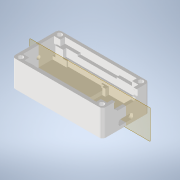
# Autodesk Inventor part: Gehäuse
Saved by Autodesk Inventor 2022 (Build 260153000, 153)
## iProperties
Created: 2021-11-08
Part Number: Gehäuse
Material: Generisch
Document SubType Name: Modeling
Designer: lukas
Density: 1 g/cm^3
Appearance: Vorgabe
Author: lukas
Autodesk Inventor part; units mm, degrees
ref_plane "YZ Plane" through (0, 0, 0) normal (1, 0, 0) x (0, 1, 0)
ref_plane "XZ Plane" through (0, 0, 0) normal (0, 1, 0) x (-1, 0, 0)
ref_plane "XY Plane" through (0, 0, 0) normal (0, 0, 1) x (1, 0, 0)
sketch "Skizze1" plane through (0, 0, 0) normal (0, 1, 0) x (-1, 0, 0)
  line L0 (0, 0) -> (58, 0)
  line L1 (58, 0) -> (58, -30)
  line L2 (58, -30) -> (0, -30)
  line L3 (0, -30) -> (0, 0)
  dimension "d0" = 30
  dimension "d1" = 58
  constraints: 8 end point, 2 parallel, 1 horizontal, 1 perpendicular
  measures "d0" distance between parallel lines of L0 L2
  measures "d1" distance of L1.end L2.end
extrude "Extrusion1" add sketch "Skizze1" along normal blind 2
sketch "Skizze2" plane through (0, 2, 0) normal (0, 1, 0) x (1, 0, 0)
  line L0 (0, 30) -> (-58, 30) projected
  line L1 (-58, 30) -> (-58, 0) projected
  line L2 (-58, 0) -> (0, 0) projected
  line L3 (0, 0) -> (0, 30) projected
  line L4 (-56, 28) -> (-2, 28)
  line L5 (-2, 28) -> (-2, 2)
  line L6 (-2, 2) -> (-56, 2)
  line L7 (-56, 2) -> (-56, 28)
  dimension "d4" = 2
  constraints: 8 end point, 3 other
  measures "d4" distance between parallel lines of L0 L4
extrude "Extrusion2" add sketch "Skizze2" along normal blind 13.7
ref_plane "Arbeitsebene1" through (-56, 2, -15) normal (0, 0, 1) x (1, 0, 0)
ref_plane "Arbeitsebene2" through (-22.61, 3.28, -21) normal (0, -1, 0) x (1, 0, 0)
sketch "Skizze6" plane through (0, 2, 0) normal (0, 1, 0) x (1, 0, 0)
  line L0 (-13, 15.5) -> (-2, 15.5) projected
  line L1 (-2, 15.5) -> (-2, 25.925) projected
  line L2 (-2, 25.925) -> (-49.2, 25.925) projected
  line L3 (-49.2, 25.925) -> (-49.2, 4.075) projected
  line L4 (-49.2, 4.075) -> (-2, 4.075) projected
  line L5 (-2, 4.075) -> (-2, 14.5) projected
  line L6 (-2, 14.5) -> (-13, 14.5) projected
  line L7 (-13, 14.5) -> (-13, 15.5) projected
  line L8 (-24.31, 7.3) -> (-24.31, 22.7) projected
  line L9 (-24.31, 22.7) -> (-17.4058, 22.7) projected
  line L10 (-17.4058, 22.7) -> (-16.0058, 21.3) projected
  line L11 (-16.0058, 21.3) -> (-7.41, 21.3) projected
  line L12 (-7.41, 8.7) -> (-16.0058, 8.7) projected
  line L13 (-16.0058, 8.7) -> (-17.4058, 7.3) projected
  line L14 (-17.4058, 7.3) -> (-24.31, 7.3) projected
  line L15 (-48.9344, 26.05) -> (-46.9344, 26.05)
  line L16 (-46.9344, 26.05) -> (-46.9344, 3.95)
  line L17 (-46.9344, 3.95) -> (-48.9344, 3.95)
  line L18 (-48.9344, 3.95) -> (-48.9344, 26.05)
  line L19 (-0.8, 14.3) -> (-11.8, 14.3)
  line L20 (-11.8, 14.3) -> (-11.8, 15.7)
  line L21 (-11.8, 15.7) -> (-0.8, 15.7)
  line L22 (-0.8, 15.7) -> (-0.8, 2.875)
  line L23 (-0.8, 2.875) -> (-50.4, 2.875)
  line L24 (-50.4, 2.875) -> (-50.4, 27.125)
  line L25 (-50.4, 27.125) -> (-0.8, 27.125)
  line L26 (-0.8, 27.125) -> (-0.8, 14.3)
  line L27 (-48.2, 24.925) -> (-3, 24.925)
  line L28 (-3, 24.925) -> (-3, 16.5)
  line L29 (-3, 16.5) -> (-14, 16.5)
  line L30 (-14, 16.5) -> (-14, 13.5)
  line L31 (-14, 13.5) -> (-3, 13.5)
  line L32 (-3, 13.5) -> (-3, 5.075)
  line L33 (-3, 5.075) -> (-48.2, 5.075)
  line L34 (-48.2, 5.075) -> (-48.2, 24.925)
  line L35 (-13.5, 6.075) -> (-13.5, 23.925) projected
  line L36 (-2, 6.075) -> (-13.5, 6.075) projected
  line L37 (-13.5, 23.925) -> (-2, 23.925) projected
  line L38 (-2, 23.925) -> (-2, 6.075) projected
  line L39 (-3, 5.075) -> (-2, 5.075)
  line L40 (-2, 2) -> (-2, 28) projected
  line L41 (-3, 24.925) -> (-2, 24.925)
  line L42 (-2, 2) -> (-2, 28) projected
  line L43 (-46.9344, 3.95) -> (-46.9344, 2.875)
  line L44 (-46.9344, 26.05) -> (-46.9344, 27.125)
  line L45 (-50.4, 27.125) -> (-46.9344, 27.125)
  line L46 (-46.9344, 27.125) -> (-46.9344, 26.25)
  line L47 (-46.9344, 26.25) -> (-50.4, 26.25)
  line L48 (-50.4, 26.25) -> (-50.4, 27.125)
  line L49 (-50.4, 2.875) -> (-46.9344, 2.875)
  line L50 (-46.9344, 2.875) -> (-46.9344, 3.75)
  line L51 (-46.9344, 3.75) -> (-50.4, 3.75)
  line L52 (-50.4, 3.75) -> (-50.4, 2.875)
  line L53 (-68, 2.495) -> (-68, 27.05)
  line L54 (-56, 28) -> (-56, 2) projected
  line L55 (-50.4, 27.125) -> (-56, 27.125)
  line L56 (-50.4, 2.875) -> (-56, 2.875)
  line L57 (-2, 28) -> (-56, 28) projected
  line L58 (-50.4, 27.125) -> (-2, 27.125)
  line L59 (-2, 27.125) -> (-2, 28)
  line L60 (-2, 28) -> (-50.4, 28)
  line L61 (-50.4, 28) -> (-50.4, 27.125)
  line L62 (-56, 2) -> (-2, 2) projected
  line L63 (-50.4, 3.75) -> (-2, 3.75)
  line L64 (-2, 3.75) -> (-2, 2)
  line L65 (-2, 2) -> (-50.4, 2)
  line L66 (-50.4, 2) -> (-50.4, 3.75)
  line L67 (-54.3, 2) -> (-49.3, 2)
  line L68 (-49.3, 2) -> (-49.3, 6)
  line L69 (-49.3, 6) -> (-54.3, 6)
  line L70 (-54.3, 6) -> (-54.3, 2)
  line L71 (-54.3, 28) -> (-49.3, 28)
  line L72 (-49.3, 28) -> (-49.3, 24)
  line L73 (-49.3, 24) -> (-54.3, 24)
  line L74 (-54.3, 24) -> (-54.3, 28)
  line L75 (-54.3, 6) -> (-46.9344, 6)
  line L76 (-46.9344, 6) -> (-46.9344, 2)
  line L77 (-46.9344, 2) -> (-54.3, 2)
  line L78 (-54.3, 2) -> (-54.3, 6)
  line L79 (-54.3, 24) -> (-46.9344, 24)
  line L80 (-46.9344, 24) -> (-46.9344, 28)
  line L81 (-46.9344, 28) -> (-54.3, 28)
  line L82 (-54.3, 28) -> (-54.3, 24)
  point P0 (0, 0)
  point P1 (-2, 11.83)
  point P2 (-2, 18.17)
  point P3 (-2, 2.875)
  point P4 (-46.9344, 5.075)
  point P5 (-46.9344, 24.925)
  point P6 (-2, 27.125)
  point P7 (-54.3, 2.875)
  point P8 (-50.4, 6)
  point P9 (-49.3, 3.75)
  point P10 (-50.4, 24)
  point P11 (-49.3, 26.25)
  point P12 (-54.3, 27.125)
  point P13 (-50.4, 24)
  point P14 (-50.4, 6)
  dimension "d26" = 2
  dimension "d27" = 1
  dimension "d53" = 0.1
  dimension "d54" = 5
  dimension "d55" = 4
  dimension "d56" = 4
  constraints: 118 end point, 19 parallel, 14 point on line, 12 perpendicular, 10 horizontal, 14 other
  measures "d26" distance of L16.end L17.end
  measures "d27" distance between parallel lines of L2 L27
  measures "d53" distance between parallel lines of L3 L68
  measures "d54" distance between parallel lines of L68 L70
  measures "d55" distance between parallel lines of L62 L69
  measures "d56" distance of L71.end L72.end
ref_plane "Arbeitsebene3" through (-49.2, 7, -25.925) normal (0, -1, 0) x (1, 0, 0)
extrude "Extrusion6" add sketch "Skizze6" along normal blind 5 contours L41 L27 L16 L2 L1 | L2 L16 L44 L25 L40 | L25 L80 L57 L40 | L5 L4 L16 L33 L39 | L16 L27 L34 L79 L18 L2 | L2 L18 L15 L16 | L16 L79 L34 L27 | L40 L62 L76 L23 | L23 L43 L63 L40 | L44 L47 L72 L25 | L25 L72 L57 L80 | L40 L63 L43 L16 L4 | L18 L79 L3 L2 | L2 L3 L79 L72 L47 L44 L15 L18 | L76 L62 L68 L23 | L23 L68 L51 L43 | L72 L47 L24 L25 | L25 L61 L57 L72 | L16 L17 L18 L4 | L4 L18 L75 L34 L33 L16 | L33 L34 L75 L16 | L68 L62 L66 L23 | L23 L24 L51 L68 | L51 L68 L75 L3 L4 L18 L17 L43 | L24 L73 L74 L55 | L55 L74 L57 L61 | L72 L73 L24 L47 | L4 L3 L75 L18 | L56 L70 L69 L24 | L66 L62 L70 L56 | L51 L24 L69 L68
sketch "Skizze9" plane through (-50.4, 7, -27.125) normal (0, 1, 0) x (1, 0, 0)
  line L0 (37.4, -11.625) -> (48.4, -11.625) projected
  line L1 (48.4, -11.625) -> (48.4, -1.2) projected
  line L2 (48.4, -1.2) -> (1.2, -1.2) projected
  line L3 (1.2, -1.2) -> (1.2, -23.05) projected
  line L4 (1.2, -23.05) -> (48.4, -23.05) projected
  line L5 (48.4, -23.05) -> (48.4, -12.625) projected
  line L6 (48.4, -12.625) -> (37.4, -12.625) projected
  line L7 (37.4, -12.625) -> (37.4, -11.625) projected
  line L8 (1.1, -1.1) -> (48.5, -1.1)
  line L9 (48.5, -1.1) -> (48.5, -11.725)
  line L10 (48.5, -11.725) -> (37.5, -11.725)
  line L11 (37.5, -11.725) -> (37.5, -12.525)
  line L12 (37.5, -12.525) -> (48.5, -12.525)
  line L13 (48.5, -12.525) -> (48.5, -23.15)
  line L14 (48.5, -23.15) -> (1.1, -23.15)
  line L15 (1.1, -23.15) -> (1.1, -1.1)
  line L16 (3.4656, -21.125) -> (-3.9, -21.125) projected
  line L17 (-3.9, -21.125) -> (-3.9, -25.125) projected
  line L18 (48.4, -25.125) -> (-3.9, -25.125) projected
  line L19 (48.4, -22.05) -> (48.4, -25.125) projected
  line L20 (48.4, -22.05) -> (3.4656, -22.05) projected
  line L21 (3.4656, -22.05) -> (3.4656, -21.125) projected
  line L22 (3.4656, -2.2) -> (48.4, -2.2) projected
  line L23 (48.4, 0.875) -> (48.4, -2.2) projected
  line L24 (-3.9, 0.875) -> (48.4, 0.875) projected
  line L25 (-3.9, 0.875) -> (-3.9, -3.125) projected
  line L26 (-3.9, -3.125) -> (3.4656, -3.125) projected
  line L27 (3.4656, -3.125) -> (3.4656, -2.2) projected
  point P0 (50.4, -27.125)
  point P1 (1.1, -3.125)
  point P2 (48.4, -1.1)
  point P3 (48.4, -23.15)
  point P4 (1.1, -21.125)
  dimension "d41" = 0.1
  constraints: 16 end point, 7 other
  measures "d41" distance between parallel lines of L2 L8
extrude "Extrusion9" add sketch "Skizze9" along normal blind 5 contours L8 L15 L26 L25 L24 L23 | L19 L18 L17 L16 L15 L14
sketch "Skizze13" plane through (-50.4, 12, -27.125) normal (0, 1, 0) x (1, 0, 0)
  line L0 (48.4, -25.125) -> (-3.9, -25.125) projected
  line L1 (48.4, -23.15) -> (48.4, -25.125) projected
  line L2 (48.4, -23.15) -> (1.1, -23.15) projected
  line L3 (1.1, -23.15) -> (1.1, -21.125) projected
  line L4 (1.1, -21.125) -> (-3.9, -21.125) projected
  line L5 (-3.9, -21.125) -> (-3.9, -25.125) projected
  line L6 (-3.9, -3.125) -> (1.1, -3.125) projected
  line L7 (1.1, -3.125) -> (1.1, -1.1) projected
  line L8 (1.1, -1.1) -> (48.4, -1.1) projected
  line L9 (48.4, 0.875) -> (48.4, -1.1) projected
  line L10 (-3.9, 0.875) -> (48.4, 0.875) projected
  line L11 (-3.9, 0.875) -> (-3.9, -3.125) projected
  line L12 (48.4, -25.125) -> (-3.9, -25.125) projected
  line L13 (48.4, -23.15) -> (1.1, -23.15) projected
  line L14 (33.4, -25.125) -> (8.4, -25.125)
  line L15 (8.4, -25.125) -> (8.4, -23.15)
  line L16 (8.4, -23.15) -> (33.4, -23.15)
  line L17 (33.4, -23.15) -> (33.4, -25.125)
  line L18 (-3.9, 0.875) -> (48.4, 0.875) projected
  line L19 (33.4, -1.1) -> (8.4, -1.1)
  line L20 (8.4, -1.1) -> (8.4, 0.875)
  line L21 (8.4, 0.875) -> (33.4, 0.875)
  line L22 (33.4, 0.875) -> (33.4, -1.1)
  point P0 (50.4, -27.125)
  point P1 (8.4, 0.875)
  point P2 (8.4, -1.1)
  point P3 (33.4, -25.125)
  point P4 (33.4, -23.15)
  point P5 (8.4, -23.15)
  point P6 (8.4, -25.125)
  dimension "d81" = 25
  dimension "d82" = 15
  constraints: 16 end point, 6 point on line, 4 parallel, 2 horizontal, 2 perpendicular
  measures "d81" distance of L15.end L16.end
  measures "d82" distance between parallel lines of L1 L17
extrude "Extrusion13" cut sketch "Skizze13" against normal blind 1 contours L0 L15 L2 L17 | L10 L22 L8 L20
sketch "Skizze14" plane through (-58, 0, -30) normal (-1, 0, 0) x (0, 0, 1)
  line L0 (0, 0) -> (30, 0) projected
  line L1 (30, 0) -> (30, 15.7) projected
  line L2 (0, 15.7) -> (30, 15.7) projected
  line L3 (0, 0) -> (0, 15.7) projected
  circle A0 centre (15, 8.7) radius 1.275
  line L4 (0, 15.7) -> (30, 15.7) projected
  point P0 (15, 15.7)
  dimension "d85" = 2.55
  dimension "d86" = 7
  constraints: 1 centre point, 1 midpoint, 1 vertical alignment
  measures "d85" diameter of A0
  measures "d86" distance from line of L2 A0.centre
extrude "Extrusion14" cut sketch "Skizze14" against normal blind 3 contours A0
sketch "Skizze15" plane through (0, 0, 0) normal (1, 0, 0) x (0, 0, -1)
  line L0 (7.5, 14.875) -> (7.5, 12.3966) projected
  arc A0 (8.3, 15.675) -> (7.5, 14.875) centre (8.3, 14.875) ccw projected
  arc A1 (7.5, 12.3966) -> (8.0647, 11.6319) centre (8.3, 12.3966) ccw projected
  line L1 (8.0647, 11.6319) -> (8.612, 11.4636) projected
  arc A2 (8.7489, 11.375) -> (8.612, 11.4636) centre (8.5237, 11.1768) ccw projected
  line L2 (8.7489, 11.375) -> (9.61, 10.3965) projected
  arc A3 (9.61, 10.3965) -> (10.2106, 10.125) centre (10.2106, 10.925) ccw projected
  line L3 (10.2106, 10.125) -> (19.7894, 10.125) projected
  arc A4 (19.7894, 10.125) -> (20.39, 10.3965) centre (19.7894, 10.925) ccw projected
  line L4 (21.2511, 11.375) -> (20.39, 10.3965) projected
  arc A5 (21.388, 11.4636) -> (21.2511, 11.375) centre (21.4763, 11.1768) ccw projected
  line L5 (21.388, 11.4636) -> (21.9353, 11.6319) projected
  arc A6 (21.9353, 11.6319) -> (22.5, 12.3966) centre (21.7, 12.3966) ccw projected
  line L6 (22.5, 12.3966) -> (22.5, 14.875) projected
  arc A7 (22.5, 14.875) -> (21.7, 15.675) centre (21.7, 14.875) ccw projected
  line L7 (8.3, 15.675) -> (21.7, 15.675) projected
  line L8 (21.229, 11.5716) -> (21.2224, 11.5696)
  line L9 (7.35, 12.3966) -> (7.35, 14.875)
  arc A8 (8.3, 15.825) -> (7.35, 14.875) centre (8.3, 14.875) ccw
  line L10 (8.3, 15.825) -> (21.7, 15.825)
  arc A9 (22.65, 14.875) -> (21.7, 15.825) centre (21.7, 14.875) ccw
  line L11 (22.65, 14.875) -> (22.65, 12.3966)
  arc A10 (21.9794, 11.4886) -> (22.65, 12.3966) centre (21.7, 12.3966) ccw
  line L12 (21.9794, 11.4886) -> (21.4322, 11.3202)
  arc A11 (21.4322, 11.3202) -> (21.3637, 11.2759) centre (21.4763, 11.1768) ccw
  line L13 (21.3637, 11.2759) -> (20.5026, 10.2974)
  arc A12 (19.7894, 9.975) -> (20.5026, 10.2974) centre (19.7894, 10.925) ccw
  line L14 (19.7894, 9.975) -> (10.2106, 9.975)
  arc A13 (9.4974, 10.2974) -> (10.2106, 9.975) centre (10.2106, 10.925) ccw
  line L15 (9.4974, 10.2974) -> (8.6363, 11.2759)
  arc A14 (8.6363, 11.2759) -> (8.5678, 11.3202) centre (8.5237, 11.1768) ccw
  line L16 (8.5678, 11.3202) -> (8.0206, 11.4886)
  arc A15 (7.35, 12.3966) -> (8.0206, 11.4886) centre (8.3, 12.3966) ccw
  point P0 (0, 0)
  dimension "d124" = 0.15
  constraints: 18 end point, 16 point on circle, 8 centre point, 15 other
  measures "d124" distance between parallel lines of L0 L9
extrude "Extrusion15" cut sketch "Skizze15" against normal blind 3 contours A0 L7 A7 L6 A6 L5 A5 L4 A4 L3 A3 L2 A2 L1 A1 L0 | L9 A8 L10 A9 L11 A10 L12 A11 L13 A12 L14 A13 L15 A14 L16 A15
sketch "Skizze17" plane through (-56, 2, -2) normal (1, 0, 0) x (0, 0, -1)
  line L0 (26, 0) -> (26, 13.7) projected
  line L1 (0, 13.7) -> (26, 13.7) projected
  line L2 (0, 0) -> (0, 13.7) projected
  line L3 (26, 0) -> (0, 0) projected
  line L4 (0, 13.7) -> (26, 13.7) projected
  line L5 (0, 13.7) -> (3, 13.7)
  line L6 (3, 13.7) -> (3, 9.5)
  line L7 (3, 9.5) -> (0, 9.5)
  line L8 (0, 9.5) -> (0, 13.7)
  line L9 (26, 4.5) -> (26, 13.7) projected
  line L10 (26, 13.7) -> (23, 13.7)
  line L11 (23, 13.7) -> (23, 9.5)
  line L12 (23, 9.5) -> (26, 9.5)
  line L13 (26, 9.5) -> (26, 13.7)
  point P0 (-2, -2)
  point P1 (26, 9.5)
  point P2 (0, 9.5)
  dimension "d98" = 3
  dimension "d99" = 4.2
  dimension "d100" = 3
  dimension "d101" = 4.2
  constraints: 16 end point, 4 parallel, 2 horizontal, 2 perpendicular
  measures "d98" distance of L6.end L7.end
  measures "d99" distance of L5.end L6.end
  measures "d100" distance of L12.end L11.end
  measures "d101" distance of L11.end L10.end
extrude "Extrusion17" add sketch "Skizze17" along normal blind 4 contours L12 L11 L1 L0 | L2 L1 L6 L7
chamfer "Fase1" distance 3 angle 45 2 edges at (-55.15, 11.5, -2) (-55.15, 11.5, -28)
sketch "Skizze18" plane through (0, 15.7, 0) normal (0, 1, 0) x (1, 0, 0)
  circle A0 centre (-3, 27.5) radius 1.6
  line L0 (0, 22.171) -> (0, 30) projected
  line L1 (0, 30) -> (-58, 30) projected
  line L2 (-58, 30) -> (-58, 0) projected
  line L3 (-58, 0) -> (0, 0) projected
  line L4 (-2, 7.829) -> (-2, 2) projected
  line L5 (-2, 2) -> (-52, 2) projected
  line L6 (-52, 5) -> (-52, 2) projected
  line L7 (-56, 5) -> (-52, 5) projected
  line L8 (-56, 5) -> (-56, 25) projected
  line L9 (-56, 25) -> (-52, 25) projected
  line L10 (-52, 28) -> (-52, 25) projected
  line L11 (-52, 28) -> (-2, 28) projected
  line L12 (0, 0) -> (0, 30) projected
  line L13 (-2, 25) -> (-6, 25) projected
  line L14 (0, 30) -> (-6, 30)
  line L15 (-6, 30) -> (-6, 25)
  line L16 (-6, 25) -> (0, 25)
  line L17 (0, 25) -> (0, 30)
  line L18 (-6, 2) -> (-6, 5) projected
  line L19 (-58, 0) -> (0, 0) projected
  line L20 (-6, 5) -> (0, 5)
  line L21 (0, 5) -> (0, 0)
  line L22 (0, 0) -> (-6, 0)
  line L23 (-6, 0) -> (-6, 5)
  circle A1 centre (-3, 2.5) radius 1.6
  circle A2 centre (-55, 27.5) radius 1.6
  circle A3 centre (-55, 2.5) radius 1.6
  line L24 (-56, 25) -> (-52, 25) projected
  line L25 (-52, 25) -> (-58, 25)
  line L26 (-58, 25) -> (-58, 30)
  line L27 (-58, 30) -> (-52, 30)
  line L28 (-52, 30) -> (-52, 25)
  line L29 (-2, 22.171) -> (0, 22.171) projected
  line L30 (0, 0) -> (0, 7.829) projected
  line L31 (0, 7.829) -> (-2, 7.829) projected
  line L32 (-2, 28) -> (-2, 22.171) projected
  point P0 (0, 22.4155)
  point P1 (-3, 25)
  point P2 (-6, 27.5)
  point P3 (-3, 5)
  point P4 (0, 2.5)
  point P5 (-55, 30)
  dimension "d107" = 3.2
  dimension "d108" = 3.2
  dimension "d109" = 3.2
  dimension "d110" = 3.2
  constraints: 24 end point, 6 parallel, 5 midpoint, 4 centre point, 4 horizontal alignment, 4 vertical alignment, 3 horizontal, 3 perpendicular
  measures "d107" diameter of A0
  measures "d108" diameter of A1
  measures "d109" diameter of A2
  measures "d110" diameter of A3
extrude "Extrusion18" cut sketch "Skizze18" against normal blind 4.05 contours A0 L32 L11 | L11 L32 A0 | A1 L5 L4 | L4 L5 A1 | A2 | A3
fillet "Rundung3" radius 2 4 edges at (0, 7.85, -30) (-58, 7.85, -30) (-58, 7.85, 0) (0, 7.85, 0)
sketch "Skizze20" plane through (0, 2, 0) normal (0, 1, 0) x (1, 0, 0)
  line L0 (-19.27, 6.05) -> (-19.27, 7.38) projected
  line L1 (-19.27, 6.05) -> (-18.73, 6.05) projected
  line L2 (-18.73, 7.38) -> (-18.73, 6.05) projected
  arc A0 (-16.73, 7.38) -> (-18.73, 7.38) centre (-17.73, 7.38) ccw projected
  line L3 (-16.73, 6.05) -> (-16.73, 7.38) projected
  line L4 (-16.73, 6.05) -> (-16.19, 6.05) projected
  line L5 (-16.19, 7.38) -> (-16.19, 6.05) projected
  arc A1 (-14.19, 7.38) -> (-16.19, 7.38) centre (-15.19, 7.38) ccw projected
  line L6 (-14.19, 6.05) -> (-14.19, 7.38) projected
  line L7 (-14.19, 6.05) -> (-13.65, 6.05) projected
  line L8 (-13.65, 7.38) -> (-13.65, 6.05) projected
  arc A2 (-11.65, 7.38) -> (-13.65, 7.38) centre (-12.65, 7.38) ccw projected
  line L9 (-11.65, 6.05) -> (-11.65, 7.38) projected
  line L10 (-11.65, 6.05) -> (-11.11, 6.05) projected
  line L11 (-11.11, 7.38) -> (-11.11, 6.05) projected
  arc A3 (-9.11, 7.38) -> (-11.11, 7.38) centre (-10.11, 7.38) ccw projected
  line L12 (-9.11, 6.05) -> (-9.11, 7.38) projected
  line L13 (-9.11, 6.05) -> (-8.57, 6.05) projected
  line L14 (-8.57, 7.38) -> (-8.57, 6.05) projected
  arc A4 (-6.57, 7.38) -> (-8.57, 7.38) centre (-7.57, 7.38) ccw projected
  line L15 (-6.57, 6.05) -> (-6.57, 7.38) projected
  line L16 (-6.57, 6.05) -> (-6.03, 6.05) projected
  line L17 (-6.03, 7.38) -> (-6.03, 6.05) projected
  arc A5 (-4.03, 7.38) -> (-6.03, 7.38) centre (-5.03, 7.38) ccw projected
  line L18 (-4.03, 6.05) -> (-4.03, 7.38) projected
  line L19 (-4.03, 6.05) -> (-2, 6.05) projected
  line L20 (-2, 6.05) -> (-2, 23.95) projected
  line L21 (-2, 23.95) -> (-4.03, 23.95) projected
  line L22 (-4.03, 22.62) -> (-4.03, 23.95) projected
  arc A6 (-6.03, 22.62) -> (-4.03, 22.62) centre (-5.03, 22.62) ccw projected
  line L23 (-6.03, 23.95) -> (-6.03, 22.62) projected
  line L24 (-6.03, 23.95) -> (-6.57, 23.95) projected
  line L25 (-6.57, 22.62) -> (-6.57, 23.95) projected
  arc A7 (-8.57, 22.62) -> (-6.57, 22.62) centre (-7.57, 22.62) ccw projected
  line L26 (-8.57, 23.95) -> (-8.57, 22.62) projected
  line L27 (-8.57, 23.95) -> (-9.11, 23.95) projected
  line L28 (-9.11, 22.62) -> (-9.11, 23.95) projected
  arc A8 (-11.11, 22.62) -> (-9.11, 22.62) centre (-10.11, 22.62) ccw projected
  line L29 (-11.11, 23.95) -> (-11.11, 22.62) projected
  line L30 (-11.11, 23.95) -> (-11.65, 23.95) projected
  line L31 (-11.65, 22.62) -> (-11.65, 23.95) projected
  arc A9 (-13.65, 22.62) -> (-11.65, 22.62) centre (-12.65, 22.62) ccw projected
  line L32 (-13.65, 23.95) -> (-13.65, 22.62) projected
  line L33 (-13.65, 23.95) -> (-14.19, 23.95) projected
  line L34 (-14.19, 22.62) -> (-14.19, 23.95) projected
  arc A10 (-16.19, 22.62) -> (-14.19, 22.62) centre (-15.19, 22.62) ccw projected
  line L35 (-16.19, 23.95) -> (-16.19, 22.62) projected
  line L36 (-16.19, 23.95) -> (-16.73, 23.95) projected
  line L37 (-16.73, 22.62) -> (-16.73, 23.95) projected
  arc A11 (-18.73, 22.62) -> (-16.73, 22.62) centre (-17.73, 22.62) ccw projected
  line L38 (-18.73, 23.95) -> (-18.73, 22.62) projected
  line L39 (-18.73, 23.95) -> (-19.27, 23.95) projected
  line L40 (-19.27, 22.62) -> (-19.27, 23.95) projected
  arc A12 (-21.27, 22.62) -> (-19.27, 22.62) centre (-20.27, 22.62) ccw projected
  line L41 (-21.27, 23.95) -> (-21.27, 22.62) projected
  line L42 (-21.27, 23.95) -> (-23.3, 23.95) projected
  line L43 (-23.3, 23.95) -> (-23.3, 6.05) projected
  line L44 (-23.3, 6.05) -> (-21.27, 6.05) projected
  line L45 (-21.27, 7.38) -> (-21.27, 6.05) projected
  arc A13 (-19.27, 7.38) -> (-21.27, 7.38) centre (-20.27, 7.38) ccw projected
  line L46 (-5.2, 8.64) -> (-5.2, 10.14) projected
  arc A14 (-5.45, 8.39) -> (-5.2, 8.64) centre (-5.45, 8.64) ccw projected
  line L47 (-6.95, 8.39) -> (-5.45, 8.39) projected
  arc A15 (-7.2, 8.64) -> (-6.95, 8.39) centre (-6.95, 8.64) ccw projected
  line L48 (-7.2, 10.14) -> (-7.2, 8.64) projected
  arc A16 (-6.95, 10.39) -> (-7.2, 10.14) centre (-6.95, 10.14) ccw projected
  line L49 (-5.45, 10.39) -> (-6.95, 10.39) projected
  arc A17 (-5.2, 10.14) -> (-5.45, 10.39) centre (-5.45, 10.14) ccw projected
  line L50 (-5.1, 10.14) -> (-5.1, 8.64) projected
  arc A18 (-4.85, 10.39) -> (-5.1, 10.14) centre (-4.85, 10.14) ccw projected
  line L51 (-3.35, 10.39) -> (-4.85, 10.39) projected
  arc A19 (-3.1, 10.14) -> (-3.35, 10.39) centre (-3.35, 10.14) ccw projected
  line L52 (-3.1, 8.64) -> (-3.1, 10.14) projected
  arc A20 (-3.35, 8.39) -> (-3.1, 8.64) centre (-3.35, 8.64) ccw projected
  line L53 (-4.85, 8.39) -> (-3.35, 8.39) projected
  arc A21 (-5.1, 8.64) -> (-4.85, 8.39) centre (-4.85, 8.64) ccw projected
  spline S0 degree 3 poles (-7.4383, 8.7265) (-7.4372, 8.7238) (-7.4352, 8.7188) (-7.4325, 8.7119) (-7.4304, 8.7061) (-7.4285, 8.7003) (-7.4269, 8.6945) (-7.4266, 8.6902) (-7.4265, 8.6883) knots 0 0 0 0 0.218644 0.402253 0.555346 0.678013 0.862007 1 1 1 1 projected
  spline S1 degree 3 poles (-7.4265, 8.6883) (-7.4265, 8.6868) (-7.4267, 8.6839) (-7.428, 8.6796) (-7.4318, 8.6761) (-7.438, 8.6737) (-7.4469, 8.6719) (-7.4563, 8.6709) (-7.4656, 8.6703) (-7.4743, 8.6703) (-7.4841, 8.6699) (-7.491, 8.67) (-7.4947, 8.67) knots 0 0 0 0 0.059095 0.112119 0.170127 0.252338 0.367432 0.521837 0.618289 0.730657 0.857328 1 1 1 1 projected
  spline S2 degree 3 poles (-7.4947, 8.67) (-7.5006, 8.6701) (-7.511, 8.6702) (-7.525, 8.6705) (-7.5358, 8.6719) (-7.544, 8.6739) (-7.5502, 8.6766) (-7.5543, 8.6806) (-7.5569, 8.6852) (-7.5582, 8.6885) (-7.5588, 8.6903) knots 0 0 0 0 0.243312 0.431629 0.577323 0.691188 0.782141 0.853383 0.924117 1 1 1 1 projected
  line L54 (-7.5588, 8.6903) -> (-7.6134, 8.8237) projected
  spline S3 degree 3 poles (-7.6134, 8.8237) (-7.6166, 8.8309) (-7.6227, 8.8445) (-7.6322, 8.8635) (-7.6419, 8.8798) (-7.653, 8.8933) (-7.6656, 8.904) (-7.6802, 8.9116) (-7.6969, 8.9163) (-7.7088, 8.9168) (-7.715, 8.9171) knots 0 0 0 0 0.159253 0.300949 0.428594 0.543395 0.652248 0.760304 0.87415 1 1 1 1 projected
  line L55 (-7.715, 8.9171) -> (-7.7529, 8.9171) projected
  line L56 (-7.7529, 8.9171) -> (-7.7529, 8.6894) projected
  spline S4 degree 3 poles (-7.7529, 8.6894) (-7.7531, 8.6879) (-7.7535, 8.6849) (-7.7559, 8.6806) (-7.7603, 8.6772) (-7.7666, 8.6747) (-7.775, 8.6728) (-7.7857, 8.6711) (-7.7993, 8.6703) (-7.8094, 8.6701) (-7.815, 8.67) knots 0 0 0 0 0.063923 0.128953 0.202861 0.29696 0.418389 0.569455 0.762357 1 1 1 1 projected
  spline S5 degree 3 poles (-7.815, 8.67) (-7.8205, 8.6701) (-7.8304, 8.6703) (-7.8439, 8.6711) (-7.8548, 8.6728) (-7.8632, 8.6747) (-7.8695, 8.6772) (-7.8737, 8.6807) (-7.8761, 8.6849) (-7.8763, 8.6879) (-7.8765, 8.6894) knots 0 0 0 0 0.235042 0.427069 0.582893 0.705011 0.797834 0.870651 0.936049 1 1 1 1 projected
  line L57 (-7.8765, 8.6894) -> (-7.8765, 9.2317) projected
  spline S6 degree 3 poles (-7.8765, 9.2317) (-7.8763, 9.2348) (-7.8761, 9.2407) (-7.8743, 9.249) (-7.8708, 9.2557) (-7.8662, 9.2611) (-7.8606, 9.2651) (-7.8543, 9.268) (-7.8474, 9.2697) (-7.8427, 9.2699) (-7.8402, 9.27) knots 0 0 0 0 0.156892 0.296423 0.417856 0.533664 0.64735 0.761616 0.877699 1 1 1 1 projected
  line L58 (-7.8402, 9.27) -> (-7.6847, 9.27) projected
  spline S7 degree 3 poles (-7.6847, 9.27) (-7.6809, 9.27) (-7.6737, 9.2701) (-7.6634, 9.2697) (-7.6542, 9.2695) (-7.6435, 9.2689) (-7.6315, 9.2682) (-7.6222, 9.2673) (-7.6178, 9.2668) knots 0 0 0 0 0.168799 0.323243 0.461226 0.582836 0.801515 1 1 1 1 projected
  spline S8 degree 3 poles (-7.6178, 9.2668) (-7.6119, 9.2659) (-7.6004, 9.264) (-7.5835, 9.2602) (-7.5676, 9.2552) (-7.5526, 9.2495) (-7.5386, 9.2427) (-7.5257, 9.2349) (-7.5137, 9.2265) (-7.5032, 9.2167) (-7.4935, 9.2062) (-7.4853, 9.1946) (-7.478, 9.1822) (-7.4721, 9.1688) (-7.4674, 9.1545) (-7.4641, 9.1391) (-7.4622, 9.1227) (-7.4619, 9.1115) (-7.4618, 9.1057) knots 0 0 0 0 0.071941 0.141275 0.208024 0.272727 0.334909 0.395041 0.453767 0.511409 0.568268 0.624997 0.682573 0.741345 0.801426 0.864331 0.930152 1 1 1 1 projected
  spline S9 degree 3 poles (-7.4618, 9.1057) (-7.4618, 9.1007) (-7.4619, 9.0911) (-7.4636, 9.0771) (-7.4658, 9.0636) (-7.4691, 9.0509) (-7.4734, 9.0388) (-7.4787, 9.0275) (-7.4848, 9.0167) (-7.4917, 9.0065) (-7.4996, 8.9972) (-7.5083, 8.9883) (-7.5178, 8.9802) (-7.5319, 8.9701) (-7.5517, 8.959) (-7.5689, 8.9529) (-7.5777, 8.9497) knots 0 0 0 0 0.070285 0.136994 0.202303 0.264733 0.325376 0.384718 0.443521 0.501618 0.559879 0.618846 0.678457 0.739139 0.866116 1 1 1 1 projected
  spline S10 degree 3 poles (-7.5777, 8.9497) (-7.5732, 8.9474) (-7.5642, 8.9429) (-7.5516, 8.9342) (-7.5396, 8.9239) (-7.5284, 8.9118) (-7.5182, 8.8976) (-7.5083, 8.8816) (-7.4989, 8.8635) (-7.4932, 8.8506) (-7.4902, 8.8439) knots 0 0 0 0 0.107803 0.215659 0.325407 0.442559 0.566569 0.69895 0.842654 1 1 1 1 projected
  line L59 (-7.4902, 8.8439) -> (-7.4383, 8.7265) projected
  spline S11 degree 3 poles (-7.6567, 10.09) (-7.6497, 10.0899) (-7.6361, 10.0898) (-7.619, 10.0887) (-7.6052, 10.0874) (-7.5941, 10.0858) (-7.5819, 10.0839) (-7.569, 10.0815) (-7.5555, 10.0784) (-7.5418, 10.0741) (-7.528, 10.0685) (-7.5142, 10.062) (-7.5009, 10.0546) (-7.4885, 10.0459) (-7.4769, 10.0366) (-7.4666, 10.0261) (-7.4573, 10.0147) (-7.4491, 10.0024) (-7.4422, 9.989) (-7.4364, 9.9749) (-7.432, 9.9597) (-7.4288, 9.9438) (-7.4269, 9.9269) (-7.4266, 9.9153) (-7.4265, 9.9094) knots 0 0 0 0 0.063007 0.123216 0.154022 0.187899 0.224828 0.264901 0.306619 0.349613 0.394249 0.440594 0.486807 0.532101 0.57657 0.620821 0.664707 0.708961 0.75382 0.799919 0.847 0.895604 0.946497 1 1 1 1 projected
  spline S12 degree 3 poles (-7.4265, 9.9094) (-7.4266, 9.9013) (-7.4269, 9.8855) (-7.4301, 9.8625) (-7.435, 9.8409) (-7.4418, 9.8208) (-7.451, 9.8022) (-7.4615, 9.785) (-7.4742, 9.7695) (-7.4884, 9.7553) (-7.5046, 9.7428) (-7.5225, 9.7321) (-7.5421, 9.7228) (-7.5634, 9.7151) (-7.5866, 9.709) (-7.6118, 9.7048) (-7.6388, 9.7022) (-7.6575, 9.7019) (-7.6672, 9.7018) knots 0 0 0 0 0.06715 0.130987 0.192023 0.250495 0.307273 0.362918 0.417933 0.473196 0.529168 0.586638 0.646152 0.708623 0.77483 0.844837 0.919909 1 1 1 1 projected
  line L60 (-7.6672, 9.7018) -> (-7.7176, 9.7018) projected
  line L61 (-7.7176, 9.7018) -> (-7.7176, 9.5096) projected
  spline S13 degree 3 poles (-7.7176, 9.5096) (-7.7178, 9.5081) (-7.7182, 9.5051) (-7.7206, 9.5008) (-7.725, 9.4974) (-7.7313, 9.4947) (-7.7397, 9.4928) (-7.7504, 9.4911) (-7.7641, 9.4903) (-7.7741, 9.4901) (-7.7797, 9.49) knots 0 0 0 0 0.063872 0.12885 0.202699 0.297519 0.418851 0.569797 0.762546 1 1 1 1 projected
  spline S14 degree 3 poles (-7.7797, 9.49) (-7.7852, 9.4901) (-7.7951, 9.4903) (-7.8086, 9.4911) (-7.8195, 9.4928) (-7.8279, 9.4947) (-7.8342, 9.4972) (-7.8384, 9.5007) (-7.8408, 9.5049) (-7.8411, 9.5079) (-7.8412, 9.5094) knots 0 0 0 0 0.235042 0.427069 0.582893 0.705011 0.797834 0.870651 0.936049 1 1 1 1 projected
  line L62 (-7.8412, 9.5094) -> (-7.8412, 10.0466) projected
  spline S15 degree 3 poles (-7.8412, 10.0466) (-7.8411, 10.05) (-7.8409, 10.0564) (-7.8386, 10.0654) (-7.8351, 10.0731) (-7.8299, 10.0793) (-7.8237, 10.0842) (-7.8164, 10.0875) (-7.8083, 10.0897) (-7.8025, 10.0899) (-7.7995, 10.09) knots 0 0 0 0 0.149716 0.282881 0.403862 0.51862 0.633697 0.747474 0.868404 1 1 1 1 projected
  line L63 (-7.7995, 10.09) -> (-7.6567, 10.09) projected
  spline S16 degree 3 poles (-2.4504, 9.27) (-2.4491, 9.2699) (-2.4463, 9.2697) (-2.4424, 9.2676) (-2.4392, 9.2641) (-2.4365, 9.259) (-2.4348, 9.2522) (-2.4332, 9.2436) (-2.4325, 9.2331) (-2.4324, 9.2254) (-2.4324, 9.2212) knots 0 0 0 0 0.070886 0.14453 0.225022 0.321454 0.442525 0.594997 0.779598 1 1 1 1 projected
  spline S17 degree 3 poles (-2.4324, 9.2212) (-2.4324, 9.2172) (-2.4325, 9.2097) (-2.4332, 9.1994) (-2.4348, 9.1911) (-2.4365, 9.1843) (-2.4392, 9.1792) (-2.4424, 9.1754) (-2.4463, 9.1734) (-2.4491, 9.1731) (-2.4504, 9.1729) knots 0 0 0 0 0.215856 0.39792 0.547509 0.670123 0.769946 0.853252 0.927835 1 1 1 1 projected
  line L64 (-2.4504, 9.1729) -> (-2.6, 9.1729) projected
  line L65 (-2.6, 9.1729) -> (-2.6, 8.6894) projected
  spline S18 degree 3 poles (-2.6, 8.6894) (-2.6002, 8.688) (-2.6006, 8.685) (-2.6029, 8.6808) (-2.6073, 8.6774) (-2.6136, 8.6747) (-2.6221, 8.6728) (-2.6329, 8.6711) (-2.6464, 8.6703) (-2.6563, 8.6701) (-2.6618, 8.67) knots 0 0 0 0 0.062311 0.127673 0.201958 0.297338 0.419387 0.573174 0.767062 1 1 1 1 projected
  spline S19 degree 3 poles (-2.6618, 8.67) (-2.6672, 8.6701) (-2.6771, 8.6703) (-2.6906, 8.6711) (-2.7014, 8.6728) (-2.7099, 8.6747) (-2.7162, 8.6774) (-2.7206, 8.6808) (-2.7232, 8.685) (-2.7234, 8.688) (-2.7235, 8.6894) knots 0 0 0 0 0.232796 0.424597 0.580239 0.702214 0.797535 0.871775 0.938071 1 1 1 1 projected
  line L66 (-2.7235, 8.6894) -> (-2.7235, 9.1729) projected
  line L67 (-2.7235, 9.1729) -> (-2.8731, 9.1729) projected
  spline S20 degree 3 poles (-2.8731, 9.1729) (-2.8746, 9.1731) (-2.8774, 9.1733) (-2.8813, 9.1755) (-2.8844, 9.1792) (-2.8868, 9.1844) (-2.8889, 9.191) (-2.8901, 9.1995) (-2.8911, 9.2097) (-2.8912, 9.2171) (-2.8912, 9.2212) knots 0 0 0 0 0.076972 0.149357 0.230988 0.32965 0.452923 0.602028 0.784232 1 1 1 1 projected
  spline S21 degree 3 poles (-2.8912, 9.2212) (-2.8912, 9.2254) (-2.8911, 9.2331) (-2.8901, 9.2436) (-2.8889, 9.2523) (-2.8868, 9.259) (-2.8844, 9.2641) (-2.8812, 9.2676) (-2.8774, 9.2698) (-2.8746, 9.2699) (-2.8731, 9.27) knots 0 0 0 0 0.22032 0.405057 0.557069 0.678794 0.774059 0.852865 0.924342 1 1 1 1 projected
  line L68 (-2.8731, 9.27) -> (-2.4504, 9.27) projected
  spline S22 degree 3 poles (-2.5218, 9.5871) (-2.5203, 9.587) (-2.5174, 9.5868) (-2.5133, 9.5847) (-2.51, 9.5811) (-2.5072, 9.5762) (-2.5053, 9.5695) (-2.5038, 9.5611) (-2.5031, 9.5508) (-2.503, 9.5433) (-2.5029, 9.5392) knots 0 0 0 0 0.078521 0.154743 0.23568 0.333831 0.453954 0.602478 0.783246 1 1 1 1 projected
  spline S23 degree 3 poles (-2.5029, 9.5392) (-2.503, 9.5351) (-2.5031, 9.5276) (-2.5038, 9.5172) (-2.5053, 9.5087) (-2.5073, 9.5018) (-2.5098, 9.4963) (-2.5132, 9.4925) (-2.5174, 9.4904) (-2.5203, 9.4901) (-2.5218, 9.49) knots 0 0 0 0 0.212451 0.39201 0.537585 0.662164 0.763554 0.847997 0.922706 1 1 1 1 projected
  line L69 (-2.5218, 9.49) -> (-2.8014, 9.49) projected
  spline S24 degree 3 poles (-2.8014, 9.49) (-2.8039, 9.4901) (-2.8088, 9.4903) (-2.8158, 9.4919) (-2.822, 9.495) (-2.8279, 9.4988) (-2.8327, 9.5041) (-2.836, 9.511) (-2.8379, 9.5193) (-2.8381, 9.5252) (-2.8382, 9.5283) knots 0 0 0 0 0.123526 0.240828 0.354113 0.467375 0.583697 0.706123 0.844455 1 1 1 1 projected
  line L70 (-2.8382, 9.5283) -> (-2.8382, 10.0706) projected
  spline S25 degree 3 poles (-2.8382, 10.0706) (-2.8381, 10.0721) (-2.8379, 10.0751) (-2.8352, 10.0792) (-2.831, 10.0828) (-2.8246, 10.0853) (-2.8161, 10.0873) (-2.8053, 10.0888) (-2.7918, 10.09) (-2.7819, 10.09) (-2.7765, 10.09) knots 0 0 0 0 0.063823 0.128372 0.203821 0.298264 0.420136 0.575648 0.767441 1 1 1 1 projected
  spline S26 degree 3 poles (-2.7765, 10.09) (-2.771, 10.09) (-2.761, 10.09) (-2.7475, 10.0889) (-2.7367, 10.0872) (-2.7284, 10.0853) (-2.722, 10.0828) (-2.7177, 10.0792) (-2.7152, 10.075) (-2.7149, 10.0721) (-2.7147, 10.0706) knots 0 0 0 0 0.236646 0.428558 0.58027 0.702218 0.796719 0.872216 0.935804 1 1 1 1 projected
  line L71 (-2.7147, 10.0706) -> (-2.7147, 9.5871) projected
  line L72 (-2.7147, 9.5871) -> (-2.5218, 9.5871) projected
  spline S27 degree 3 poles (-2.1296, 20.8) (-2.1281, 20.7999) (-2.1251, 20.7997) (-2.1209, 20.7974) (-2.1174, 20.7936) (-2.1145, 20.7881) (-2.1126, 20.7807) (-2.1109, 20.7714) (-2.1102, 20.76) (-2.1101, 20.7517) (-2.11, 20.7471) knots 0 0 0 0 0.070886 0.14453 0.225022 0.321454 0.442525 0.594997 0.779598 1 1 1 1 projected
  spline S28 degree 3 poles (-2.11, 20.7471) (-2.1101, 20.7427) (-2.1102, 20.7347) (-2.1109, 20.7236) (-2.1126, 20.7145) (-2.1145, 20.7071) (-2.1174, 20.7016) (-2.1209, 20.6976) (-2.1251, 20.6953) (-2.1281, 20.695) (-2.1296, 20.6949) knots 0 0 0 0 0.215856 0.39792 0.547509 0.670123 0.769946 0.853252 0.927835 1 1 1 1 projected
  line L73 (-2.1296, 20.6949) -> (-2.2916, 20.6949) projected
  line L74 (-2.2916, 20.6949) -> (-2.2916, 20.1711) projected
  spline S29 degree 3 poles (-2.2916, 20.1711) (-2.2918, 20.1695) (-2.2922, 20.1663) (-2.2948, 20.1617) (-2.2996, 20.158) (-2.3064, 20.1551) (-2.3155, 20.153) (-2.3272, 20.1512) (-2.3419, 20.1503) (-2.3527, 20.1501) (-2.3585, 20.15) knots 0 0 0 0 0.062311 0.127673 0.201958 0.297338 0.419387 0.573174 0.767062 1 1 1 1 projected
  spline S30 degree 3 poles (-2.3585, 20.15) (-2.3644, 20.1501) (-2.3751, 20.1503) (-2.3898, 20.1512) (-2.4015, 20.153) (-2.4107, 20.1551) (-2.4175, 20.158) (-2.4222, 20.1617) (-2.425, 20.1662) (-2.4253, 20.1695) (-2.4254, 20.1711) knots 0 0 0 0 0.232796 0.424597 0.580239 0.702214 0.797535 0.871775 0.938071 1 1 1 1 projected
  line L75 (-2.4254, 20.1711) -> (-2.4254, 20.6949) projected
  line L76 (-2.4254, 20.6949) -> (-2.5875, 20.6949) projected
  spline S31 degree 3 poles (-2.5875, 20.6949) (-2.5891, 20.695) (-2.5921, 20.6953) (-2.5964, 20.6976) (-2.5997, 20.7016) (-2.6023, 20.7072) (-2.6046, 20.7144) (-2.6059, 20.7236) (-2.607, 20.7347) (-2.607, 20.7427) (-2.6071, 20.7471) knots 0 0 0 0 0.076972 0.149357 0.230988 0.32965 0.452923 0.602028 0.784232 1 1 1 1 projected
  spline S32 degree 3 poles (-2.6071, 20.7471) (-2.607, 20.7517) (-2.607, 20.76) (-2.6059, 20.7714) (-2.6046, 20.7808) (-2.6023, 20.788) (-2.5997, 20.7936) (-2.5963, 20.7974) (-2.5921, 20.7998) (-2.5891, 20.7999) (-2.5875, 20.8) knots 0 0 0 0 0.22032 0.405057 0.557069 0.678794 0.774059 0.852865 0.924342 1 1 1 1 projected
  line L77 (-2.5875, 20.8) -> (-2.1296, 20.8) projected
  spline S33 degree 3 poles (-2.9885, 20.6378) (-2.9883, 20.6343) (-2.9881, 20.6275) (-2.9858, 20.6177) (-2.9818, 20.6087) (-2.9765, 20.6004) (-2.9698, 20.5928) (-2.9621, 20.5856) (-2.9535, 20.5787) (-2.9401, 20.5703) (-2.9216, 20.5602) (-2.8973, 20.5494) (-2.8714, 20.5386) (-2.8449, 20.527) (-2.8182, 20.5145) (-2.7922, 20.5002) (-2.7676, 20.4837) (-2.7496, 20.467) (-2.7367, 20.4523) (-2.7282, 20.4402) (-2.7206, 20.4272) (-2.7138, 20.4133) (-2.7083, 20.3982) (-2.7045, 20.3818) (-2.702, 20.3642) (-2.7018, 20.3519) (-2.7017, 20.3457) knots 0 0 0 0 0.023878 0.046244 0.068492 0.090674 0.113592 0.137421 0.162608 0.188939 0.245122 0.30648 0.370814 0.436937 0.504051 0.572129 0.639419 0.706115 0.739403 0.772825 0.807138 0.84229 0.878452 0.916579 0.957095 1 1 1 1 projected
  spline S34 degree 3 poles (-2.7017, 20.3457) (-2.7019, 20.3374) (-2.7023, 20.3214) (-2.7059, 20.2981) (-2.7121, 20.2763) (-2.7204, 20.2561) (-2.7312, 20.2377) (-2.7435, 20.2208) (-2.7574, 20.2054) (-2.7733, 20.1918) (-2.7906, 20.1797) (-2.8094, 20.1692) (-2.8295, 20.1604) (-2.8509, 20.1531) (-2.8734, 20.1474) (-2.8968, 20.1435) (-2.9209, 20.1408) (-2.9373, 20.1406) (-2.9456, 20.1404) knots 0 0 0 0 0.068777 0.134078 0.196814 0.25728 0.316408 0.374537 0.432005 0.489854 0.548758 0.608405 0.669363 0.732297 0.797125 0.863039 0.930856 1 1 1 1 projected
  spline S35 degree 3 poles (-2.9456, 20.1404) (-2.9566, 20.1407) (-2.9778, 20.1411) (-3.0082, 20.1454) (-3.0356, 20.1517) (-3.0598, 20.1588) (-3.0803, 20.1667) (-3.0971, 20.1752) (-3.1098, 20.1833) (-3.1197, 20.1905) (-3.126, 20.1996) (-3.1289, 20.2088) (-3.1303, 20.2178) (-3.1312, 20.2262) (-3.1318, 20.2359) (-3.1318, 20.2428) (-3.1318, 20.2465) knots 0 0 0 0 0.135706 0.262615 0.379538 0.483083 0.574416 0.65187 0.715307 0.761317 0.802014 0.850154 0.879538 0.91425 0.954388 1 1 1 1 projected
  spline S36 degree 3 poles (-3.1318, 20.2465) (-3.1318, 20.2514) (-3.1317, 20.2603) (-3.131, 20.2725) (-3.1298, 20.2824) (-3.1277, 20.2901) (-3.1252, 20.2962) (-3.1215, 20.3003) (-3.117, 20.3025) (-3.1138, 20.3028) (-3.1121, 20.3029) knots 0 0 0 0 0.223135 0.407876 0.557255 0.677647 0.775427 0.852758 0.924021 1 1 1 1 projected
  spline S37 degree 3 poles (-3.1121, 20.3029) (-3.1108, 20.3028) (-3.1078, 20.3025) (-3.103, 20.3006) (-3.0975, 20.2978) (-3.0887, 20.2921) (-3.0756, 20.2838) (-3.0568, 20.2735) (-3.0341, 20.2631) (-3.0124, 20.2555) (-2.993, 20.2504) (-2.9769, 20.2476) (-2.9597, 20.2459) (-2.9478, 20.2457) (-2.9417, 20.2456) knots 0 0 0 0 0.022334 0.04925 0.083285 0.123704 0.221109 0.338658 0.475249 0.631298 0.715846 0.80477 0.8993 1 1 1 1 projected
  spline S38 degree 3 poles (-2.9417, 20.2456) (-2.9339, 20.2459) (-2.9189, 20.2464) (-2.8977, 20.2507) (-2.8793, 20.2577) (-2.8636, 20.2669) (-2.8511, 20.2791) (-2.842, 20.2937) (-2.8365, 20.3106) (-2.8358, 20.3225) (-2.8355, 20.3286) knots 0 0 0 0 0.154687 0.296231 0.424785 0.542153 0.653407 0.764721 0.879462 1 1 1 1 projected
  spline S39 degree 3 poles (-2.8355, 20.3286) (-2.8356, 20.3322) (-2.8359, 20.3391) (-2.8384, 20.3491) (-2.8423, 20.3583) (-2.85, 20.3694) (-2.8626, 20.382) (-2.881, 20.3951) (-2.9025, 20.4068) (-2.9266, 20.4175) (-2.9525, 20.4283) (-2.9791, 20.4398) (-3.0058, 20.4525) (-3.0318, 20.4668) (-3.0562, 20.4833) (-3.0741, 20.4999) (-3.087, 20.5146) (-3.0956, 20.5268) (-3.1033, 20.5399) (-3.11, 20.554) (-3.1157, 20.5693) (-3.1195, 20.586) (-3.1219, 20.6042) (-3.1222, 20.6168) (-3.1223, 20.6233) knots 0 0 0 0 0.024103 0.0471 0.069243 0.09169 0.138868 0.189533 0.244856 0.305167 0.369196 0.435316 0.502565 0.570024 0.636717 0.702619 0.735749 0.769486 0.803636 0.838927 0.87567 0.914275 0.955607 1 1 1 1 projected
  spline S40 degree 3 poles (-3.1223, 20.6233) (-3.1221, 20.6308) (-3.1218, 20.6455) (-3.1184, 20.6667) (-3.1129, 20.6866) (-3.105, 20.7049) (-3.0955, 20.7218) (-3.0843, 20.7373) (-3.0714, 20.7511) (-3.0572, 20.7635) (-3.0415, 20.7746) (-3.0244, 20.7839) (-3.0061, 20.7921) (-2.9864, 20.7983) (-2.9659, 20.8034) (-2.9446, 20.807) (-2.9227, 20.8091) (-2.908, 20.8094) (-2.9005, 20.8096) knots 0 0 0 0 0.069191 0.134511 0.19726 0.257963 0.317406 0.375727 0.433059 0.490802 0.548962 0.608581 0.669649 0.733194 0.798249 0.864168 0.931303 1 1 1 1 projected
  spline S41 degree 3 poles (-2.9005, 20.8096) (-2.8926, 20.8094) (-2.8768, 20.8091) (-2.8535, 20.8059) (-2.8309, 20.8016) (-2.8098, 20.7958) (-2.7905, 20.789) (-2.7762, 20.7825) (-2.7662, 20.7771) (-2.7603, 20.7736) (-2.7557, 20.7704) (-2.7516, 20.7667) (-2.7483, 20.7627) (-2.7452, 20.7584) (-2.7435, 20.7537) (-2.7419, 20.7483) (-2.741, 20.7415) (-2.7402, 20.7333) (-2.7401, 20.723) (-2.74, 20.7156) (-2.7399, 20.7114) knots 0 0 0 0 0.109619 0.220032 0.327445 0.429538 0.524488 0.611357 0.649203 0.681543 0.706931 0.727544 0.757548 0.780046 0.800902 0.826805 0.857694 0.895982 0.942453 1 1 1 1 projected
  spline S42 degree 3 poles (-2.7399, 20.7114) (-2.7399, 20.7069) (-2.74, 20.6985) (-2.7405, 20.687) (-2.7416, 20.6775) (-2.7428, 20.6698) (-2.7451, 20.6639) (-2.7481, 20.6594) (-2.7526, 20.657) (-2.7558, 20.6567) (-2.7576, 20.6566) knots 0 0 0 0 0.215054 0.397257 0.547048 0.669861 0.766401 0.845802 0.918791 1 1 1 1 projected
  spline S43 degree 3 poles (-2.7576, 20.6566) (-2.7587, 20.6567) (-2.7612, 20.6569) (-2.7653, 20.6587) (-2.7702, 20.6611) (-2.7783, 20.6658) (-2.7903, 20.6727) (-2.8068, 20.6814) (-2.8263, 20.6898) (-2.8443, 20.6963) (-2.8602, 20.7004) (-2.8729, 20.7028) (-2.8863, 20.7042) (-2.8954, 20.7043) (-2.9, 20.7044) knots 0 0 0 0 0.021788 0.050042 0.08603 0.12997 0.23501 0.357907 0.498098 0.652959 0.735072 0.820912 0.908692 1 1 1 1 projected
  spline S44 degree 3 poles (-2.9, 20.7044) (-2.907, 20.7043) (-2.9202, 20.704) (-2.9384, 20.6999) (-2.9538, 20.6941) (-2.9665, 20.686) (-2.9767, 20.6762) (-2.9833, 20.6643) (-2.9878, 20.6514) (-2.9882, 20.6424) (-2.9885, 20.6378) knots 0 0 0 0 0.168147 0.315376 0.446752 0.564837 0.675062 0.78304 0.89035 1 1 1 1 projected
  spline S45 degree 3 poles (-3.2584, 20.2112) (-3.2572, 20.2083) (-3.255, 20.2029) (-3.2521, 20.1954) (-3.2499, 20.1891) (-3.2478, 20.1828) (-3.2461, 20.1765) (-3.2457, 20.1719) (-3.2456, 20.1699) knots 0 0 0 0 0.218644 0.402253 0.555346 0.678013 0.862007 1 1 1 1 projected
  spline S46 degree 3 poles (-3.2456, 20.1699) (-3.2457, 20.1682) (-3.2458, 20.1651) (-3.2472, 20.1604) (-3.2514, 20.1566) (-3.2581, 20.154) (-3.2677, 20.1521) (-3.2779, 20.1509) (-3.288, 20.1503) (-3.2974, 20.1504) (-3.308, 20.1499) (-3.3155, 20.15) (-3.3195, 20.15) knots 0 0 0 0 0.059095 0.112119 0.170127 0.252338 0.367432 0.521837 0.618289 0.730657 0.857328 1 1 1 1 projected
  spline S47 degree 3 poles (-3.3195, 20.15) (-3.3259, 20.1501) (-3.3372, 20.1502) (-3.3523, 20.1506) (-3.364, 20.1521) (-3.3729, 20.1542) (-3.3796, 20.1572) (-3.3841, 20.1615) (-3.3869, 20.1665) (-3.3883, 20.1701) (-3.389, 20.172) knots 0 0 0 0 0.243312 0.431629 0.577323 0.691188 0.782141 0.853383 0.924117 1 1 1 1 projected
  line L78 (-3.389, 20.172) -> (-3.4481, 20.3165) projected
  spline S48 degree 3 poles (-3.4481, 20.3165) (-3.4516, 20.3243) (-3.4582, 20.3391) (-3.4684, 20.3596) (-3.479, 20.3773) (-3.491, 20.392) (-3.5046, 20.4035) (-3.5205, 20.4118) (-3.5386, 20.4169) (-3.5514, 20.4174) (-3.5582, 20.4176) knots 0 0 0 0 0.159253 0.300949 0.428594 0.543395 0.652248 0.760304 0.87415 1 1 1 1 projected
  line L79 (-3.5582, 20.4176) -> (-3.5993, 20.4176) projected
  line L80 (-3.5993, 20.4176) -> (-3.5993, 20.1711) projected
  spline S49 degree 3 poles (-3.5993, 20.1711) (-3.5995, 20.1694) (-3.5999, 20.1662) (-3.6024, 20.1615) (-3.6072, 20.1578) (-3.6141, 20.1551) (-3.6231, 20.153) (-3.6348, 20.1512) (-3.6495, 20.1503) (-3.6605, 20.1501) (-3.6665, 20.15) knots 0 0 0 0 0.063923 0.128953 0.202861 0.29696 0.418389 0.569455 0.762357 1 1 1 1 projected
  spline S50 degree 3 poles (-3.6665, 20.15) (-3.6724, 20.1501) (-3.6832, 20.1503) (-3.6978, 20.1512) (-3.7096, 20.153) (-3.7187, 20.1551) (-3.7255, 20.1578) (-3.7301, 20.1616) (-3.7327, 20.1662) (-3.733, 20.1694) (-3.7331, 20.1711) knots 0 0 0 0 0.235042 0.427069 0.582893 0.705011 0.797834 0.870651 0.936049 1 1 1 1 projected
  line L81 (-3.7331, 20.1711) -> (-3.7331, 20.7585) projected
  spline S51 degree 3 poles (-3.7331, 20.7585) (-3.7329, 20.7619) (-3.7327, 20.7683) (-3.7307, 20.7772) (-3.727, 20.7845) (-3.722, 20.7903) (-3.7159, 20.7947) (-3.7091, 20.7979) (-3.7016, 20.7997) (-3.6965, 20.7999) (-3.6938, 20.8) knots 0 0 0 0 0.156892 0.296423 0.417856 0.533664 0.64735 0.761616 0.877699 1 1 1 1 projected
  line L82 (-3.6938, 20.8) -> (-3.5253, 20.8) projected
  spline S52 degree 3 poles (-3.5253, 20.8) (-3.5213, 20.8) (-3.5134, 20.8001) (-3.5023, 20.7997) (-3.4923, 20.7995) (-3.4807, 20.7988) (-3.4677, 20.798) (-3.4577, 20.797) (-3.4529, 20.7966) knots 0 0 0 0 0.168799 0.323243 0.461226 0.582836 0.801515 1 1 1 1 projected
  spline S53 degree 3 poles (-3.4529, 20.7966) (-3.4465, 20.7955) (-3.434, 20.7935) (-3.4157, 20.7894) (-3.3985, 20.7839) (-3.3822, 20.7778) (-3.367, 20.7704) (-3.3531, 20.762) (-3.3401, 20.7528) (-3.3287, 20.7422) (-3.3182, 20.7309) (-3.3093, 20.7184) (-3.3014, 20.7049) (-3.2951, 20.6903) (-3.2899, 20.6748) (-3.2864, 20.6582) (-3.2843, 20.6404) (-3.284, 20.6282) (-3.2838, 20.622) knots 0 0 0 0 0.071941 0.141275 0.208024 0.272727 0.334909 0.395041 0.453767 0.511409 0.568268 0.624997 0.682573 0.741345 0.801426 0.864331 0.930152 1 1 1 1 projected
  spline S54 degree 3 poles (-3.2838, 20.622) (-3.2839, 20.6166) (-3.284, 20.6062) (-3.2858, 20.591) (-3.2882, 20.5764) (-3.2918, 20.5626) (-3.2964, 20.5495) (-3.3022, 20.5372) (-3.3087, 20.5256) (-3.3162, 20.5146) (-3.3248, 20.5044) (-3.3342, 20.4948) (-3.3446, 20.486) (-3.3598, 20.4751) (-3.3812, 20.4631) (-3.3999, 20.4565) (-3.4094, 20.453) knots 0 0 0 0 0.070285 0.136994 0.202303 0.264733 0.325376 0.384718 0.443521 0.501618 0.559879 0.618846 0.678457 0.739139 0.866116 1 1 1 1 projected
  spline S55 degree 3 poles (-3.4094, 20.453) (-3.4045, 20.4506) (-3.3948, 20.4456) (-3.3811, 20.4362) (-3.3681, 20.4251) (-3.3561, 20.4119) (-3.3449, 20.3965) (-3.3342, 20.3792) (-3.3241, 20.3596) (-3.3179, 20.3456) (-3.3146, 20.3383) knots 0 0 0 0 0.107803 0.215659 0.325407 0.442559 0.566569 0.69895 0.842654 1 1 1 1 projected
  line L83 (-3.3146, 20.3383) -> (-3.2584, 20.2112) projected
  circle A22 centre (-6.5, 20.45) radius 0.65 projected
  circle A23 centre (-4.5, 20.45) radius 0.6 projected
  line L84 (-23.5, 24.15) -> (-2, 24.15)
  line L85 (-2, 24.15) -> (-2, 5.85)
  line L86 (-2, 5.85) -> (-23.5, 5.85)
  line L87 (-23.5, 5.85) -> (-23.5, 24.15)
  line L88 (-2, 24.925) -> (-46.9344, 24.925) projected
  line L89 (-46.9344, 24.925) -> (-46.9344, 24) projected
  line L90 (-46.9344, 24) -> (-54.3, 24) projected
  line L91 (-54.3, 24) -> (-54.3, 28) projected
  line L92 (-54.3, 28) -> (-56, 28) projected
  line L93 (-56, 28) -> (-56, 2) projected
  line L94 (-56, 2) -> (-54.3, 2) projected
  line L95 (-54.3, 2) -> (-54.3, 6) projected
  line L96 (-54.3, 6) -> (-46.9344, 6) projected
  line L97 (-46.9344, 6) -> (-46.9344, 5.075) projected
  line L98 (-46.9344, 5.075) -> (-2, 5.075) projected
  line L99 (-2, 5.075) -> (-2, 24.925) projected
  line L100 (-2, 24.925) -> (-46.9344, 24.925) projected
  line L101 (-24.5, 24.925) -> (-24.5, 5.075)
  line L102 (-2, 5.075) -> (-46.9344, 5.075) projected
  point P0 (0, 0)
  point P1 (-2, 24.15)
  point P2 (-2, 5.85)
  dimension "d117" = 0.2
  dimension "d118" = 0.2
  dimension "d119" = 0.2
  dimension "d121" = 1
  constraints: 10 end point, 2 parallel, 2 perpendicular, 2 point on line, 1 horizontal, 1 vertical alignment
  measures "d117" distance between parallel lines of L42 L84
  measures "d118" distance between parallel lines of L44 L86
  measures "d119" distance between parallel lines of L43 L87
  measures "d121" distance between parallel lines of L101 L87
extrude "Extrusion20" add sketch "Skizze20" along normal blind 1 contours L99 L98 L101 L88 L84 L87 L86
